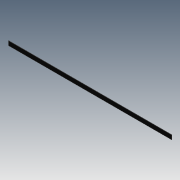
# Autodesk Inventor part: GE-12078-01
Saved by Autodesk Inventor 2012 (Build 160160000, 160)
## iProperties
Created: 2011-11-28
Part Number: GE-12078-01
Document SubType Name: Modeling
Designer: dfoster
Density: 1 g/cm^3
Description: 1" Velcro Hook, Adhesive Backed
Material: Default
Title: 1" Velcro Hook, Adhesive Backed
Author: dfoster
Autodesk Inventor part; units mm, degrees
ref_plane "YZ Plane" through (0, 0, 0) normal (1, 0, 0) x (0, 1, 0)
ref_plane "XZ Plane" through (0, 0, 0) normal (0, 1, 0) x (-1, 0, 0)
ref_plane "XY Plane" through (0, 0, 0) normal (0, 0, 1) x (1, 0, 0)
sketch "Sketch1" plane through (0, 0, 0) normal (0, 0, 1) x (1, 0, 0)
  line L0 (0, 0) -> (-977.9, 0)
  line L1 (-977.9, 0) -> (-977.9, 25.4)
  line L2 (-977.9, 25.4) -> (0, 25.4)
  line L3 (0, 25.4) -> (0, 0)
  dimension "d0" = 977.9
  dimension "d1" = 25.4
  constraints: 8 end point, 2 horizontal, 2 vertical
  measures "d0" distance of L1.end L2.end
  measures "d1" distance of L2.end L0.start
extrude "Extrusion1" add sketch "Sketch1" along normal blind 1.5875
body "Solid1"
